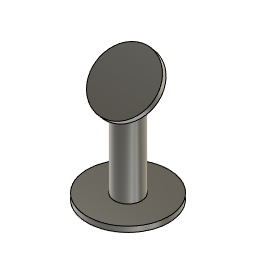
putkifinalkansi (Autodesk Fusion 360 design; units mm, degrees)
Autodesk Fusion 360 part; units mm, degrees
cylinder "CylinderPrimitive1" add diameter 20 height 80 placed x (1, 0, 0) y (0, 1, 0) z (0, 0, 1) at (0, 0, 0) makes body 1
hole "Hole1" at (0, 0, 80) direction (0, 0, -1) diameter 16 depth 80 tip angle 118 bodies 1
sketch "Sketch2" plane through (0, 0, 0) normal (1, 0, 0) x (0, 1, 0)
  line L0 (10, 80) -> (-10, 63)
surface "Extrude1" add extruded along (1, 0, 0) between -13 and 13 path "Sketch2" along L0 separate body makes body 2
extrude "Extrude2" cut 1 faces at (-4.3333, 3.3333, 74.3333) along direction (0, -0.647648, 0.761939) blind 17 on bodies 2 bodies 1
delete_face "SurfaceDeleteFace1" leaving the opening 1 faces at (-4.3333, 3.3333, 74.3333) on bodies 2
hole "Hole2" at (0, 10, 59.9954) direction (0, -1, 0) diameter 8 depth 13 tip angle 118 bodies 1
cylinder "CylinderPrimitive2" add diameter 20 height 6 placed x (1, 0, 0) y (0, 1, 0) z (0, 0, 1) at (0, 0, 0) bodies 1
sketch "Sketch4" plane through (0, 0, 0) normal (0, 0, 1) x (1, 0, 0)
  line L0 (-2.47, -1.5) -> (2.5, -1.5)
  line L1 (2.5, -1.5) -> (2.5, 1.65)
  line L2 (2.5, 1.65) -> (-2.47, 1.65)
  line L3 (-2.47, 1.65) -> (-2.47, -1.5)
  dimension "d15" = 4.97
  dimension "d16" = 3.15
  constraint horizontal L0
  constraint perpendicular L0 L1
  constraint perpendicular L1 L2
  constraint perpendicular L0 L3
  measures "d15" distance of L0.start L0.end
  measures "d16" distance of L0.end L1.end
extrude "Extrude3" cut sketch "Sketch4" along normal blind 50 bodies 1
sketch "Sketch5" plane through (0, 0, 0) normal (0, 0, 1) x (1, 0, 0)
  circle A0 centre (0, 0) radius 8
  line L0 (-7.4546, 2.9034) -> (7.4546, 2.9034)
  dimension "d19" = 16
  constraint coincident A0.centre origin
  constraint coincident A0 L0.start
  constraint coincident A0 L0.end
  constraint horizontal L0
  measures "d19" diameter of A0
extrude "Extrude4" cut sketch "Sketch5" along normal blind 50 contours A0 L0 picked at (1.817, 3.8874) bodies 1
cylinder "CylinderPrimitive3" add diameter 60 height -2 placed x (1, 0, 0) y (0, 1, 0) z (0, 0, 1) at (0, 0, 0) bodies 1
hole "Hole3" at (0, 0, -2) direction (0, 0, 1) diameter 16 depth 2 tip angle 180 bodies 1
extrude "Extrude5" add 1 faces at (23.1844, -1.9872, 0) along direction (0, 0, 1) blind 2 on bodies 1 bodies 1
cylinder "CylinderPrimitive4" add diameter 44.616 height 4 placed x (1, 0, 0) y (0, 0.761939, 0.647648) z (0, -0.647648, 0.761939) at (0, 0, 71.5) bodies 1
